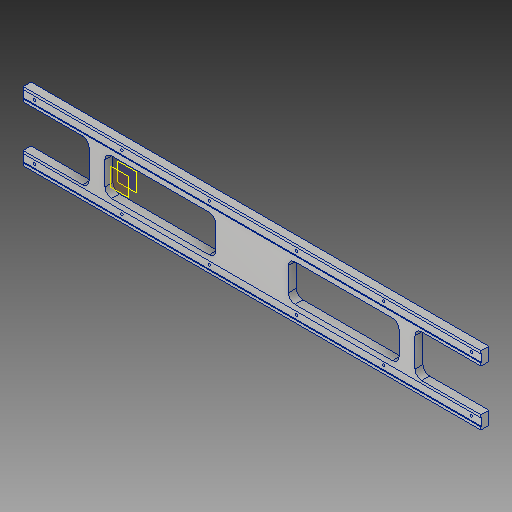
# Autodesk Inventor part: 1021topDT
Saved by Autodesk Inventor 2017 (Build 210142000, 142)
## iProperties
Created: 2016-10-15
Part Number: 1021topDT
Material: Aluminum 6061
Document SubType Name: Modeling
Designer: Kevin G
Density: 2.7 g/cm^3
Appearance: Aluminum - Flat
Author: Kevin G
Autodesk Inventor part; units mm, degrees
ref_plane "YZ Plane" through (0, 0, 0) normal (1, 0, 0) x (0, 1, 0)
ref_plane "XZ Plane" through (0, 0, 0) normal (0, 1, 0) x (-1, 0, 0)
ref_plane "XY Plane" through (0, 0, 0) normal (0, 0, 1) x (1, 0, 0)
sketch "Sketch1" plane through (0, 0, 0) normal (0, 0, 1) x (1, 0, 0)
  line L0 (-115.57, 41.275) -> (435.2925, 41.275)
  line L1 (435.2925, -41.275) -> (-115.57, -41.275)
  line L2 (422, 41.275) -> (422, 25.4)
  line L3 (424, -41.275) -> (424, -25.4)
  line L4 (355.9175, 17.4) -> (355.9175, -17.4)
  line L5 (355.9175, 6) -> (336.8675, 6)
  line L6 (321, 41.275) -> (321, 22.225)
  line L7 (322, -41.275) -> (322, -22.225)
  line L8 (336.8675, 14.225) -> (336.8675, -14.225)
  line L9 (-36.195, -17.4) -> (-36.195, 17.4)
  line L10 (-36.195, 0) -> (-17.145, 0)
  line L11 (-17.145, 14.225) -> (-17.145, -14.225)
  line L12 (-9.145, -22.225) -> (108.205, -22.225)
  line L13 (116.205, -14.225) -> (116.205, 14.225)
  line L14 (108.205, 22.225) -> (-9.145, 22.225)
  line L15 (116.205, 12) -> (203.518, 12)
  line L16 (211.518, 22.225) -> (328.8675, 22.225)
  line L17 (203.518, 14.225) -> (203.518, -14.225)
  line L18 (211.518, -22.225) -> (328.8675, -22.225)
  arc A0 (-9.145, 22.225) -> (-17.145, 14.225) centre (-9.145, 14.225) ccw
  arc A1 (116.205, 14.225) -> (108.205, 22.225) centre (108.205, 14.225) ccw
  arc A2 (-17.145, -14.225) -> (-9.145, -22.225) centre (-9.145, -14.225) ccw
  arc A3 (108.205, -22.225) -> (116.205, -14.225) centre (108.205, -14.225) ccw
  arc A4 (211.518, 22.225) -> (203.518, 14.225) centre (211.518, 14.225) ccw
  arc A5 (336.8675, 14.225) -> (328.8675, 22.225) centre (328.8675, 14.225) ccw
  arc A6 (328.8675, -22.225) -> (336.8675, -14.225) centre (328.8675, -14.225) ccw
  arc A7 (203.518, -14.225) -> (211.518, -22.225) centre (211.518, -14.225) ccw
  arc A8 (363.9175, 25.4) -> (355.9175, 17.4) centre (363.9175, 17.4) ccw
  arc A9 (355.9175, -17.4) -> (363.9175, -25.4) centre (363.9175, -17.4) ccw
  arc A10 (-36.195, 17.4) -> (-44.195, 25.4) centre (-44.195, 17.4) ccw
  arc A11 (-44.195, -25.4) -> (-36.195, -17.4) centre (-44.195, -17.4) ccw
  line L19 (435.2925, -41.275) -> (435.2925, 38.1)
  line L20 (-115.57, 41.275) -> (-115.57, -38.1)
  line L21 (-44.195, 25.4) -> (-115.57, 25.4)
  line L22 (-44.195, -25.4) -> (-115.57, -25.4)
  line L23 (363.9175, 25.4) -> (435.2925, 25.4)
  line L24 (363.9175, -25.4) -> (435.2925, -25.4)
  line L25 (-115.57, -38.1) -> (-115.57, -41.275)
  line L26 (435.2925, 41.275) -> (435.2925, 38.1)
  point P0 (0, 0)
  point P1 (-36.195, 25.4)
  point P2 (154, 41.275)
  point P3 (157.175, 41.275)
  point P4 (154, -41.275)
  point P5 (157.175, -41.275)
  dimension "d2" = 15.875
  dimension "d3" = 15.875
  dimension "d7" = 19.05
  dimension "d8" = 19.05
  dimension "d9" = 19.05
  dimension "d12" = 19.05
  dimension "d13" = 44.45
  dimension "d14" = 133.35
  dimension "d19" = 87.313
  dimension "d20" = 133.3495
  dimension "d21" = 8
  dimension "d34" = 79.375
  dimension "d35" = 79.375
  dimension "d113" = 550.8625
  constraints: 54 end point, 24 point on circle, 20 tangent, 15 point on line, 12 centre point, 11 equal radius, 9 perpendicular, 8 vertical, 5 horizontal, 2 parallel, 1 midpoint
  measures "d2" distance of L2.start L2.end
  measures "d3" distance of L3.end L3.start
  measures "d7" distance of L5.start L5.end
  measures "d8" distance of L6.start L6.end
  measures "d9" distance of L7.end L7.start
  measures "d12" distance of L10.start L10.end
  measures "d13" distance between parallel lines of L12 L14
  measures "d14" distance between parallel lines of L13 L11
  measures "d19" distance of L15.end L15.start
  measures "d20" distance between parallel lines of L8 L17
  measures "d21" radius of A0
  measures "d34" distance between parallel lines of L19 L4
  measures "d35" distance between parallel lines of L20 L9
  measures "d113" distance of L0.start L0.end
ref_plane "Work Plane2" through (0, 0, 9.525) normal (0, 0, 1) x (1, 0, 0)
sketch "Sketch2" plane through (0, 0, 9.525) normal (0, 0, 1) x (1, 0, 0)
  line L0 (-115.57, 41.275) -> (154, 41.275) projected
  line L1 (-71.7405, 41.275) -> (-71.7405, 38.1)
  line L2 (-44.195, 25.4) -> (-115.57, 25.4) projected
  line L3 (-83, 25.4) -> (-83, 28.575)
  line L4 (154, -41.275) -> (-130.57, -41.275) projected
  line L5 (-85, -41.275) -> (-85, -38.1)
  line L6 (-115.57, -25.4) -> (-44.195, -25.4) projected
  line L7 (-76, -25.4) -> (-76, -28.575)
  line L8 (-115.57, 25.4) -> (-115.57, 41.275) projected
  line L9 (435.2925, 25.4) -> (435.2925, 38.1) projected
  line L10 (-115.57, 38.1) -> (435.2925, 38.1)
  line L11 (435.2925, 38.1) -> (435.2925, 28.575)
  line L12 (435.2925, 28.575) -> (-115.57, 28.575)
  line L13 (-115.57, 28.575) -> (-115.57, 38.1)
  line L14 (-115.57, -38.1) -> (-115.57, -25.4) projected
  line L15 (435.2925, -25.4) -> (435.2925, -41.275) projected
  line L16 (-115.57, -28.575) -> (435.2925, -28.575)
  line L17 (435.2925, -28.575) -> (435.2925, -38.1)
  line L18 (435.2925, -38.1) -> (-115.57, -38.1)
  line L19 (-115.57, -38.1) -> (-115.57, -28.575)
  point P0 (0, 0)
  dimension "d39" = 3.175
  dimension "d40" = 3.175
  dimension "d41" = 3.175
  dimension "d42" = 3.175
  constraints: 24 end point, 8 point on line, 4 parallel, 3 perpendicular, 3 vertical, 2 horizontal
  measures "d39" distance of L1.start L1.end
  measures "d40" distance of L3.end L3.start
  measures "d41" distance of L5.end L5.start
  measures "d42" distance of L7.start L7.end
ref_plane "Work Plane1" through (0, 0, 0) normal (0, 0, -1) x (-1, 0, 0)
sketch "Sketch4" plane through (0, 0, 0) normal (0, 0, -1) x (-1, 0, 0)
  line L0 (-435.2925, 87) -> (-422.5925, 87)
  line L1 (-435.2925, -87) -> (-422.5925, -87)
  line L2 (-422.5925, 114) -> (102.87, 114)
  line L3 (102.87, 99) -> (115.57, 99)
  line L4 (102.87, -91) -> (115.57, -91)
  line L5 (-422.5925, 106) -> (-317.5, 106)
  line L6 (-317.5, 90) -> (-212.4075, 90)
  line L7 (-212.4075, 109) -> (-107.315, 109)
  line L8 (-107.315, 90) -> (-2.2225, 90)
  circle A0 centre (-317.5, 33.3375) radius 3.175
  circle A1 centre (-317.5, -33.3375) radius 3.175
  circle A2 centre (-422.5925, 33.3375) radius 3.175
  circle A3 centre (-422.5925, -33.3375) radius 3.175
  circle A4 centre (-212.4075, 33.3375) radius 3.175
  circle A5 centre (-107.315, 33.3375) radius 3.175
  circle A6 centre (-2.2225, 33.3375) radius 3.175
  circle A7 centre (102.87, 33.3375) radius 3.175
  circle A8 centre (-212.4075, -33.3375) radius 3.175
  circle A9 centre (-107.315, -33.3375) radius 3.175
  circle A10 centre (-2.2225, -33.3375) radius 3.175
  circle A11 centre (102.87, -33.3375) radius 3.175
  point P0 (0, 0)
  dimension "d67" = 12.7
  dimension "d68" = 12.7
  dimension "d69" = 525.4625
  dimension "d70" = 12.7
  dimension "d71" = 105.0925
  dimension "d72" = 105.0925
  dimension "d73" = 105.0925
  dimension "d74" = 105.0925
  dimension "d75" = 105.0925
  dimension "d76" = 6.35
  dimension "d77" = 6.35
  dimension "d78" = 6.35
  dimension "d79" = 6.35
  dimension "d80" = 6.35
  dimension "d81" = 6.35
  dimension "d82" = 6.35
  dimension "d83" = 6.35
  dimension "d84" = 6.35
  dimension "d85" = 6.35
  dimension "d86" = 6.35
  dimension "d87" = 6.35
  constraints: 18 end point, 12 centre point, 9 horizontal
  measures "d67" distance of L0.start L0.end
  measures "d68" distance of L1.start L1.end
  measures "d69" distance of L2.end L2.start
  measures "d70" distance of L4.start L4.end
  measures "d71" distance of L5.start L5.end
  measures "d72" distance of L6.start L6.end
  measures "d73" distance of L7.start L7.end
  measures "d74" distance of L8.end L8.start
  measures "d75" horizontal distance of L3.start L8.end
  measures "d76" diameter of A0
  measures "d77" diameter of A2
  measures "d78" diameter of A3
  measures "d79" diameter of A4
  measures "d80" diameter of A1
  measures "d81" diameter of A8
  measures "d82" diameter of A5
  measures "d83" diameter of A9
  measures "d84" diameter of A6
  measures "d85" diameter of A10
  measures "d86" diameter of A7
  measures "d87" diameter of A11
extrude "Extrusion2" add sketch "Sketch1" along normal blind 9.525 contours L0 L6 L16 A4 L17 L15 L13 A1 L14 A0 L11 L10 L9 A10 L21 L20 | L0 L2 L23 A8 L4 L5 L8 A5 L16 L6 | L0 L26 L19 L23 L2 | L22 A11 L9 L10 L11 A2 L12 A3 L13 L15 L17 A7 L18 L7 L1 L25 L20 | L19 L1 L3 L24 | L5 L4 A9 L24 L3 L1 L7 L18 A6 L8
emboss "Emboss2" sketch "Sketch2" operation cut depth 1 direction (0, 0, -1) contours L10 L9 L12 L8 | L16 L15 L18 L14
hole "Hole3" at (-102.87, -33.3375, 0) at (2.2225, -33.3375, 0) at (107.315, -33.3375, 0) at (212.4075, -33.3375, 0) at (317.5, -33.3375, 0) at (422.5925, -33.3375, 0) at (-102.87, 33.3375, 0) at (2.2225, 33.3375, 0) at (107.315, 33.3375, 0) at (212.4075, 33.3375, 0) at (317.5, 33.3375, 0) at (422.5925, 33.3375, 0) direction (0, 0, 1) diameter 3 end through all countersink diameter 4 countersink angle 90
body "Solid1"
